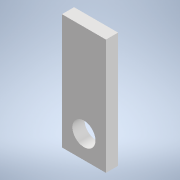
# Autodesk Inventor part: Part6
Saved by Autodesk Inventor 2022 (Build 260153000, 153)
## iProperties
Created: 2023-01-03
Part Number: Part6
Material: Generic
Document SubType Name: Modeling
Designer: Kamil
Density: 1 g/cm^3
Appearance: Default
Author: Kamil
Autodesk Inventor part; units mm, degrees
ref_plane "YZ Plane" through (0, 0, 0) normal (1, 0, 0) x (0, 1, 0)
ref_plane "XZ Plane" through (0, 0, 0) normal (0, 1, 0) x (-1, 0, 0)
ref_plane "XY Plane" through (0, 0, 0) normal (0, 0, 1) x (1, 0, 0)
sketch "Sketch1" plane through (0, 0, 0) normal (0, 0, 1) x (1, 0, 0)
  line L0 (3.625, -9.5) -> (-3.625, -9.5) projected
  line L1 (3.625, 9.5) -> (3.625, -9.5) projected
  line L2 (-3.625, 9.5) -> (3.625, 9.5) projected
  line L3 (-3.625, -9.5) -> (-3.625, 9.5) projected
  circle A0 centre (0, -5.75) radius 1.8997 projected
  circle A1 centre (0, -5.75) radius 1.9
  point P0 (0, 0)
  dimension "d0" = 3.8
  constraints: 1 centre point, 1 coincident
  measures "d0" diameter of A1
extrude "Extrusion1" add sketch "Sketch1" along normal blind 2
body "Solid1"
